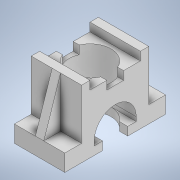
# Autodesk Inventor part: Деталь2
Saved by Autodesk Inventor 2021.2 (Build 252289000, 289)
## iProperties
Created: 2023-10-06
Part Number: Деталь2
Material: Типовые
Document SubType Name: Modeling
Designer: User
Density: 1 g/cm^3
Appearance: По умолчанию
Author: User
Autodesk Inventor part; units mm, degrees
ref_plane "YZ Plane" through (0, 0, 0) normal (1, 0, 0) x (0, 1, 0)
ref_plane "XZ Plane" through (0, 0, 0) normal (0, 1, 0) x (-1, 0, 0)
ref_plane "XY Plane" through (0, 0, 0) normal (0, 0, 1) x (1, 0, 0)
sketch "Эскиз1" plane through (0, 0, 0) normal (0, 1, 0) x (-1, 0, 0)
  line L0 (30, 60) -> (-30, 60)
  line L1 (-30, 60) -> (-30, -60)
  line L2 (-30, -60) -> (30, -60)
  line L3 (30, -60) -> (30, 60)
  point P0 (0, 0)
  dimension "d0" = 60
  dimension "d1" = 120
  constraints: 8 end point, 2 parallel, 1 horizontal, 1 perpendicular
  measures "d0" distance of L2.end L1.end
  measures "d1" distance of L1.end L0.end
extrude "Выдавливание1" add sketch "Эскиз1" along normal blind 80
sketch "Эскиз2" plane through (0, 0, 0) normal (1, 0, 0) x (0, 1, 0)
  line L0 (80, 60) -> (80, -60) projected
  line L1 (80, -30) -> (70, -30)
  line L2 (80, -30) -> (90, -30) construction
  line L3 (70, -30) -> (70, -10)
  line L4 (70, -10) -> (60, -10)
  line L5 (60, -10) -> (60, 10)
  line L6 (60, 10) -> (70, 10)
  line L7 (70, 10) -> (70, 30)
  line L8 (70, 30) -> (80, 30)
  constraints: 16 end point, 5 perpendicular, 4 point on line, 1 collinear, 1 horizontal, 1 vertical
extrude "Выдавливание2" cut sketch "Эскиз2" against normal mid plane 80
sketch "Эскиз3" plane through (0, 0, 0) normal (1, 0, 0) x (0, 1, 0)
  line L0 (0, 60) -> (0, -60) projected
  line L1 (0, -15) -> (10, -15)
  line L2 (0, -15) -> (10, -15) construction
  line L3 (10, -15) -> (10, -25)
  line L4 (10, -25) -> (15, -25)
  line L5 (0, -15) -> (0, 15)
  line L6 (0, 15) -> (10, 15)
  line L7 (10, 15) -> (10, 25)
  line L8 (10, 25) -> (15, 25)
  arc A0 (15, -25) -> (15, 25) centre (15, 0) ccw
  point P0 (0, 0)
  dimension "d20" = 10
  dimension "d21" = 0
  dimension "d22" = 30
  constraints: 16 end point, 6 perpendicular, 2 point on circle, 2 point on line, 1 centre point, 1 collinear, 1 horizontal
  measures "d20" distance of L1.start L1.end
  measures "d21" distance between parallel lines of L1 L2
  measures "d22" distance of L1.start L5.end
extrude "Выдавливание3" cut sketch "Эскиз3" against normal mid plane 80
sketch "Эскиз4" plane through (0, 0, 0) normal (0, 1, 0) x (-1, 0, 0)
  circle A0 centre (0, 0) radius 25
  dimension "d25" = 50
  constraints: 1 centre point, 1 coincident
  measures "d25" diameter of A0
extrude "Выдавливание4" cut sketch "Эскиз4" along normal blind 80
sketch "Эскиз5" plane through (30, 0, -60) normal (1, 0, 0) x (0, 0, -1)
  line L0 (-120, 0) -> (-120, 80) projected
  line L1 (-120, 20) -> (-100, 20)
  line L2 (-120, 20) -> (-100, 20) construction
  line L3 (-100, 20) -> (-100, 80)
  line L4 (-120, 80) -> (-90, 80) projected
  line L5 (0, 0) -> (0, 80) projected
  line L6 (0, 20) -> (-20, 20)
  line L7 (0, 20) -> (20, 20) construction
  line L8 (-20, 20) -> (-20, 80)
  line L9 (0, 80) -> (-30, 80) projected
  point P0 (-60, 0)
  dimension "d28" = 20
  dimension "d29" = 0
  dimension "d30" = 20
  dimension "d31" = 180
  constraints: 12 end point, 4 perpendicular, 4 point on line, 2 collinear, 2 horizontal
  measures "d28" distance of L1.start L1.end
  measures "d29" distance between parallel lines of L1 L2
  measures "d30" distance of L6.start L6.end
  measures "d31" angle of L6 L7
extrude "Выдавливание5" cut sketch "Эскиз5" against normal blind 25
sketch "Эскиз6" plane through (-30, 0, 60) normal (-1, 0, 0) x (0, 0, 1)
  line L0 (-120, 0) -> (-120, 80) projected
  line L1 (-120, 20) -> (-100, 20) projected
  line L2 (-120, 20) -> (-100, 20)
  line L3 (-100, 20) -> (-100, 80)
  line L4 (-120, 80) -> (-90, 80) projected
  line L5 (-20, 20) -> (0, 20) projected
  line L6 (0, 20) -> (-20, 20)
  line L7 (-20, 80) -> (-20, 20) projected
  line L8 (-20, 20) -> (-20, 80)
  line L9 (-20, 80) -> (-30, 80) projected
  line L10 (-30, 80) -> (0, 80) projected
  line L11 (-20, 80) -> (0, 80)
  line L12 (0, 20) -> (0, 80) projected
  line L13 (0, 80) -> (0, 20)
  point P0 (-60, 0)
  constraints: 12 end point, 3 collinear, 2 horizontal, 2 point on line, 1 perpendicular
extrude "Выдавливание6" cut sketch "Эскиз6" against normal blind 25
sketch "Эскиз7" plane through (5, 0, -60) normal (1, 0, 0) x (0, 0, -1)
  line L0 (-20, 80) -> (-20, 20) projected
  line L1 (-20, 20) -> (0, 20) projected
  line L2 (-20, 80) -> (0, 20)
  line L3 (0, 20) -> (-20, 20)
  line L4 (0, 80) -> (-20, 80) projected
  line L5 (-20, 20) -> (-20, 80)
  line L6 (0, 20) -> (0, 80) projected
  line L7 (0, 80) -> (0, 20)
  point P0 (-60, 0)
  constraints: 8 end point, 1 collinear, 1 perpendicular, 1 vertical
extrude "Выдавливание7" cut sketch "Эскиз7" against normal blind 25 contours L4 L6 L2
sketch "Эскиз8" plane through (5, 0, -60) normal (1, 0, 0) x (0, 0, -1)
  line L0 (-120, 20) -> (-120, 80) projected
  line L1 (-100, 80) -> (-120, 20)
  line L2 (-120, 20) -> (-120, 80)
  line L3 (-120, 80) -> (-100, 80) projected
  line L4 (-120, 80) -> (-100, 80)
  point P0 (-60, 0)
  constraints: 6 end point, 2 collinear
extrude "Выдавливание8" cut sketch "Эскиз8" against normal blind 25
